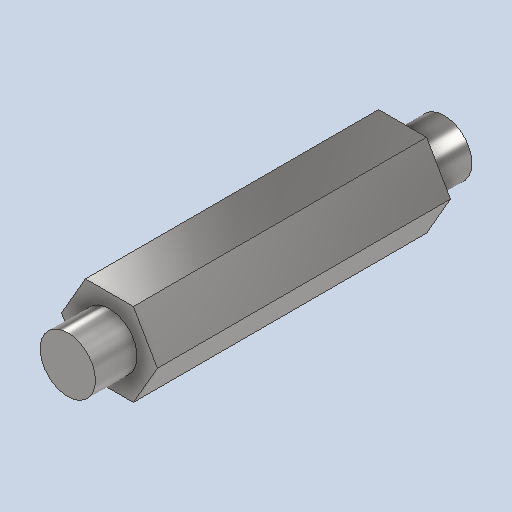
# Autodesk Inventor part: CH-1-01-motorShaft
Saved by Autodesk Inventor 2025.1 (Build 291241020, 241B)
## iProperties
Created: 2022-11-08
Part Number: CH-1-01-motorShaft
Material: Steel, Alloy
Document SubType Name: Modeling
Designer: megan
Density: 7.73 g/cm^3
Appearance: Semi-Polished
Mass: 8.0785 g
Surface Area: 7.21659 cm^2
Volume: 1.04508 cm^3
Author: megan
Autodesk Inventor part; units mm, degrees
ref_plane "YZ Plane" through (0, 0, 0) normal (1, 0, 0) x (0, 1, 0)
ref_plane "XZ Plane" through (0, 0, 0) normal (0, 1, 0) x (-1, 0, 0)
ref_plane "XY Plane" through (0, 0, 0) normal (0, 0, 1) x (1, 0, 0)
sketch "Sketch1" plane through (0, 0, 0) normal (0, 0, 1) x (1, 0, 0)
  circle A0 centre (0, 0) radius 3.175
  line L0 (2.7496, 4.7625) -> (5.4993, 0)
  line L1 (5.4993, 0) -> (2.7496, -4.7625)
  line L2 (2.7496, -4.7625) -> (-2.7496, -4.7625)
  line L3 (-2.7496, -4.7625) -> (-5.4993, 0)
  line L4 (-5.4993, 0) -> (-2.7496, 4.7625)
  line L5 (-2.7496, 4.7625) -> (2.7496, 4.7625)
  dimension "d0" = 6.35
  dimension "d3" = 9.525
  constraints: 12 end point, 2 coincident, 1 centre point, 1 horizontal, 13 other
  measures "d0" diameter of A0
  measures "d3" distance between parallel lines of L5 L2
extrude "Extrusion1" add sketch "Sketch1" along normal mid plane 43.18 contours A0
extrude "Extrusion2" add sketch "Sketch1" along normal mid plane 33.6296 contours A0 | L0 L1 L2 L3 L4 L5
body "Solid1"
